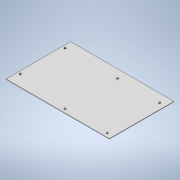
# Autodesk Inventor part: MotherboardPlate
Saved by Autodesk Inventor 2021 (Build 250183000, 183)
## iProperties
Created: 2022-01-09
Part Number: MotherboardPlate
Material: Generic
Document SubType Name: Modeling
Designer: ipodk
Density: 1 g/cm^3
Appearance: Default
Author: ipodk
Autodesk Inventor part; units mm, degrees
ref_plane "YZ Plane" through (0, 0, 0) normal (1, 0, 0) x (0, 1, 0)
ref_plane "XZ Plane" through (0, 0, 0) normal (0, 1, 0) x (-1, 0, 0)
ref_plane "XY Plane" through (0, 0, 0) normal (0, 0, 1) x (1, 0, 0)
sketch "Sketch1" plane through (0, 0, 0) normal (0, 1, 0) x (-1, 0, 0)
  line L0 (0, 0) -> (304.8, 0)
  line L1 (304.8, 0) -> (304.8, -190.5)
  line L2 (304.8, -190.5) -> (0, -190.5)
  line L3 (0, -190.5) -> (0, 0)
  dimension "d0" = 304.8
  dimension "d1" = 190.5
  constraints: 8 end point, 2 parallel, 1 horizontal, 1 perpendicular
  measures "d0" distance of L1.end L2.end
  measures "d1" distance of L0.end L1.end
extrude "Extrusion1" add sketch "Sketch1" along normal blind 1.6
sketch "Sketch2" plane through (0, 1.6, 0) normal (0, 1, 0) x (1, 0, 0)
  line L0 (-304.8, 0) -> (0, 0) projected
  line L1 (-140.97, 0) -> (-140.97, 10.16)
  line L2 (-140.97, 0) -> (-130.81, 0) construction
  line L3 (-140.97, 10.16) -> (-140.97, 33.02)
  line L4 (-140.97, 33.02) -> (-255.8376, 33.02)
  line L5 (-140.97, 10.16) -> (-95.25, 10.16)
  line L6 (-95.25, 10.16) -> (-16.51, 10.16)
  line L7 (-16.51, 10.16) -> (-16.51, 165.1)
  line L8 (-140.97, 10.16) -> (-140.97, 165.1)
  line L9 (0, 0) -> (0, 190.5) projected
  line L10 (-16.51, 165.1) -> (-295.91, 165.1)
  line L11 (-295.91, 165.1) -> (-295.91, 33.02)
  line L12 (-295.91, 33.02) -> (-255.8376, 33.02)
  circle A0 centre (-295.91, 33.02) radius 2.54
  circle A1 centre (-295.91, 165.1) radius 2.54
  circle A2 centre (-140.97, 165.1) radius 2.54
  circle A3 centre (-16.51, 165.1) radius 2.54
  circle A4 centre (-16.51, 10.16) radius 2.54
  circle A5 centre (-140.97, 10.16) radius 2.54
  point P0 (-299.72, 0)
  point P1 (-5.08, 0)
  point P2 (0, 5.08)
  point P3 (0, 185.42)
  dimension "d5" = 10.16
  dimension "d6" = 90
  dimension "d8" = 78.74
  dimension "d9" = 45.72
  dimension "d10" = 22.86
  dimension "d11" = 154.94
  dimension "d12" = 154.94
  dimension "d13" = 16.51
  dimension "d14" = 279.4
  dimension "d15" = 5.08
  dimension "d16" = 5.08
  dimension "d17" = 5.08
  dimension "d18" = 5.08
  dimension "d19" = 5.08
  dimension "d20" = 5.08
  constraints: 22 end point, 6 centre point, 6 coincident, 4 horizontal, 4 perpendicular, 3 point on line, 2 vertical
  measures "d5" distance of L1.start L1.end
  measures "d6" angle of L2 L1
  measures "d8" distance of L5.end L6.end
  measures "d9" distance of L1.end L5.end
  measures "d10" distance of L1.end L3.end
  measures "d11" distance of L6.end L7.end
  measures "d12" distance of L1.end L8.end
  measures "d13" distance between parallel lines of L7 L9
  measures "d14" distance of L7.end L10.end
  measures "d15" diameter of A0
  measures "d16" diameter of A1
  measures "d17" diameter of A2
  measures "d18" diameter of A5
  measures "d19" diameter of A4
  measures "d20" diameter of A3
extrude "Extrusion2" cut sketch "Sketch2" against normal through all contours A5 L3 L1 | L1 L5 A5 | L3 A5 L5 | A2 L10 L8 | L8 L10 A2 | A4 L7 L6 | L6 L7 A4 | A0 L11 L12 | L12 L11 A0 | L10 A2 | A1 L11 L10 | L10 L11 A1 | A3 L7 L10 | L10 L7 A3
sketch "Sketch3" plane through (0, 0, 0) normal (0, 1, 0) x (-1, 0, 0)
  circle A0 centre (16.51, -165.1) radius 2.54 projected
  circle A1 centre (16.51, -165.1) radius 2.3813
  circle A2 centre (16.51, -10.16) radius 2.54 projected
  circle A3 centre (16.51, -10.16) radius 2.3813
  circle A4 centre (140.97, -10.16) radius 2.54 projected
  circle A5 centre (140.97, -10.16) radius 2.3813
  circle A6 centre (295.91, -33.02) radius 2.54 projected
  circle A7 centre (295.91, -33.02) radius 2.3813
  circle A8 centre (295.91, -165.1) radius 2.54 projected
  circle A9 centre (295.91, -165.1) radius 2.3813
  circle A10 centre (140.97, -165.1) radius 2.54 projected
  circle A11 centre (140.97, -165.1) radius 2.3813
  point P0 (0, 0)
  constraints: 6 centre point, 6 coincident
extrude "Extrusion3" add sketch "Sketch3" along normal blind 2.54 contours A0 | A1 | A2 | A3 | A4 | A5 | A6 | A7 | A8 | A9 | A10 | A11
sketch "Sketch4" plane through (-140.97, 2.54, -10.16) normal (0, 1, 0) x (1, 0, 0)
  circle A0 centre (0, 0) radius 1.9812
  circle A1 centre (-154.94, 22.86) radius 2.54 projected
  circle A2 centre (-154.94, 22.86) radius 1.9812
  circle A3 centre (0, 154.94) radius 2.54 projected
  circle A4 centre (0, 154.94) radius 1.9812
  circle A5 centre (124.46, 154.94) radius 2.54 projected
  circle A6 centre (124.46, 154.94) radius 1.9812
  circle A7 centre (-154.94, 154.94) radius 2.54 projected
  circle A8 centre (-154.94, 154.94) radius 1.9812
  circle A9 centre (124.46, 0) radius 2.54 projected
  circle A10 centre (124.46, 0) radius 1.9812
  point P0 (140.97, -10.16)
  dimension "d25" = 3.9624
  dimension "d26" = 3.9624
  dimension "d27" = 3.9624
  dimension "d28" = 3.9624
  dimension "d29" = 3.9624
  constraints: 6 centre point, 5 coincident
  measures "d25" diameter of A0
  measures "d26" diameter of A2
  measures "d27" diameter of A4
  measures "d28" diameter of A8
  measures "d29" diameter of A10
extrude "Extrusion4" add sketch "Sketch4" along normal blind 1.27 contours A0 | A2 | A4 | A6 | A8 | A10
equation "\"d12\" = d11"
equation "\"d16\" = d15"
equation "\"d17\" = d15"
equation "\"d18\" = d15"
equation "\"d19\" = d15"
equation "\"d20\" = d15"
body "Solid1"
